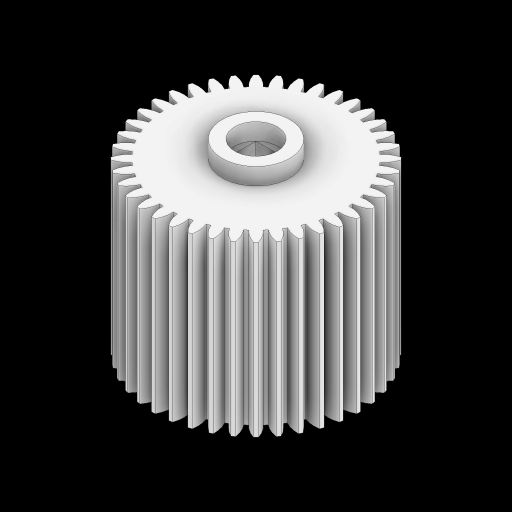
# Autodesk Inventor part: 피니언기어
Saved by Autodesk Inventor 2023 (Build 270158000, 158)
## iProperties
Created: 2024-07-04
Part Number: 피니언기어
Material: 일반
Document SubType Name: Modeling
Designer: OMS55
Density: 1 g/cm^3
Appearance: 기본값
Mass: 14.1026 g
Surface Area: 70.7702 cm^2
Volume: 14.1026 cm^3
Author: OMS55
Autodesk Inventor part; units mm, degrees
ref_plane "YZ Plane" through (0, 0, 0) normal (1, 0, 0) x (0, 1, 0)
ref_plane "XZ Plane" through (0, 0, 0) normal (0, 1, 0) x (-1, 0, 0)
ref_plane "XY Plane" through (0, 0, 0) normal (0, 0, 1) x (1, 0, 0)
sketch "스케치1" plane through (0, 0, 0) normal (0, 1, 0) x (-1, 0, 0)
  circle A0 centre (0, 0) radius 15.2
  arc A1 (12.978, 0.7559) -> (12.978, -0.7559) centre (0, 0) ccw
  line L0 (15.2, 0) -> (-15.2, 0) construction
  line L1 (15.1743, 0.8838) -> (-15.1743, -0.8838) construction
  line L2 (15.0972, 1.7646) -> (-15.0972, -1.7646) construction
  line L3 (14.9691, 2.6395) -> (-14.9691, -2.6395) construction
  line L4 (14.7903, 3.5054) -> (-14.7903, -3.5054) construction
  line L5 (14.5614, 4.3594) -> (-14.5614, -4.3594) construction
  line L6 (14.2833, 5.1987) -> (-14.2833, -5.1987) construction
  line L7 (13.9569, 6.0204) -> (-13.9569, -6.0204) construction
  line L8 (13.5832, 6.8217) -> (-13.5832, -6.8217) construction
  line L9 (13.1636, 7.6) -> (-13.1636, -7.6) construction
  line L10 (12.6994, 8.3525) -> (-12.6994, -8.3525) construction
  line L11 (12.1923, 9.0768) -> (-12.1923, -9.0768) construction
  line L12 (11.6439, 9.7704) -> (-11.6439, -9.7704) construction
  line L13 (11.0561, 10.4309) -> (-11.0561, -10.4309) construction
  line L14 (10.4309, 11.0561) -> (-10.4309, -11.0561) construction
  line L15 (9.7704, 11.6439) -> (-9.7704, -11.6439) construction
  line L16 (9.0768, 12.1923) -> (-9.0768, -12.1923) construction
  line L17 (8.3525, 12.6994) -> (-8.3525, -12.6994) construction
  line L18 (7.6, 13.1636) -> (-7.6, -13.1636) construction
  line L19 (6.8217, 13.5832) -> (-6.8217, -13.5832) construction
  line L20 (6.0204, 13.9569) -> (-6.0204, -13.9569) construction
  line L21 (5.1987, 14.2833) -> (-5.1987, -14.2833) construction
  line L22 (4.3594, 14.5614) -> (-4.3594, -14.5614) construction
  line L23 (3.5054, 14.7903) -> (-3.5054, -14.7903) construction
  line L24 (2.6395, 14.9691) -> (-2.6395, -14.9691) construction
  line L25 (1.7646, 15.0972) -> (-1.7646, -15.0972) construction
  line L26 (0.8838, 15.1743) -> (-0.8838, -15.1743) construction
  line L27 (0, 15.2) -> (0, -15.2) construction
  line L28 (-0.8838, 15.1743) -> (0.8838, -15.1743) construction
  line L29 (-1.7646, 15.0972) -> (1.7646, -15.0972) construction
  line L30 (-2.6395, 14.9691) -> (2.6395, -14.9691) construction
  line L31 (-3.5054, 14.7903) -> (3.5054, -14.7903) construction
  line L32 (-4.3594, 14.5614) -> (4.3594, -14.5614) construction
  line L33 (-5.1987, 14.2833) -> (5.1987, -14.2833) construction
  line L34 (-6.0204, 13.9569) -> (6.0204, -13.9569) construction
  line L35 (-6.8217, 13.5832) -> (6.8217, -13.5832) construction
  line L36 (-7.6, 13.1636) -> (7.6, -13.1636) construction
  line L37 (-8.3525, 12.6994) -> (8.3525, -12.6994) construction
  line L38 (-9.0768, 12.1923) -> (9.0768, -12.1923) construction
  line L39 (-9.7704, 11.6439) -> (9.7704, -11.6439) construction
  line L40 (-10.4309, 11.0561) -> (10.4309, -11.0561) construction
  line L41 (-11.0561, 10.4309) -> (11.0561, -10.4309) construction
  line L42 (-11.6439, 9.7704) -> (11.6439, -9.7704) construction
  line L43 (-12.1923, 9.0768) -> (12.1923, -9.0768) construction
  line L44 (-12.6994, 8.3525) -> (12.6994, -8.3525) construction
  line L45 (-13.1636, 7.6) -> (13.1636, -7.6) construction
  line L46 (-13.5832, 6.8217) -> (13.5832, -6.8217) construction
  line L47 (-13.9569, 6.0204) -> (13.9569, -6.0204) construction
  line L48 (-14.2833, 5.1987) -> (14.2833, -5.1987) construction
  line L49 (-14.5614, 4.3594) -> (14.5614, -4.3594) construction
  line L50 (-14.7903, 3.5054) -> (14.7903, -3.5054) construction
  line L51 (-14.9691, 2.6395) -> (14.9691, -2.6395) construction
  line L52 (-15.0972, 1.7646) -> (15.0972, -1.7646) construction
  line L53 (-15.1743, 0.8838) -> (15.1743, -0.8838) construction
  line L54 (-15.2, 0) -> (15.2, 0) construction
  line L55 (-15.1743, -0.8838) -> (15.1743, 0.8838) construction
  line L56 (-15.0972, -1.7646) -> (15.0972, 1.7646) construction
  line L57 (-14.9691, -2.6395) -> (14.9691, 2.6395) construction
  line L58 (-14.7903, -3.5054) -> (14.7903, 3.5054) construction
  line L59 (-14.5614, -4.3594) -> (14.5614, 4.3594) construction
  line L60 (-14.2833, -5.1987) -> (14.2833, 5.1987) construction
  line L61 (-13.9569, -6.0204) -> (13.9569, 6.0204) construction
  line L62 (-13.5832, -6.8217) -> (13.5832, 6.8217) construction
  line L63 (-13.1636, -7.6) -> (13.1636, 7.6) construction
  line L64 (-12.6994, -8.3525) -> (12.6994, 8.3525) construction
  line L65 (-12.1923, -9.0768) -> (12.1923, 9.0768) construction
  line L66 (-11.6439, -9.7704) -> (11.6439, 9.7704) construction
  line L67 (-11.0561, -10.4309) -> (11.0561, 10.4309) construction
  line L68 (-10.4309, -11.0561) -> (10.4309, 11.0561) construction
  line L69 (-9.7704, -11.6439) -> (9.7704, 11.6439) construction
  line L70 (-9.0768, -12.1923) -> (9.0768, 12.1923) construction
  line L71 (-8.3525, -12.6994) -> (8.3525, 12.6994) construction
  line L72 (-7.6, -13.1636) -> (7.6, 13.1636) construction
  line L73 (-6.8217, -13.5832) -> (6.8217, 13.5832) construction
  line L74 (-6.0204, -13.9569) -> (6.0204, 13.9569) construction
  line L75 (-5.1987, -14.2833) -> (5.1987, 14.2833) construction
  line L76 (-4.3594, -14.5614) -> (4.3594, 14.5614) construction
  line L77 (-3.5054, -14.7903) -> (3.5054, 14.7903) construction
  line L78 (-2.6395, -14.9691) -> (2.6395, 14.9691) construction
  line L79 (-1.7646, -15.0972) -> (1.7646, 15.0972) construction
  line L80 (-0.8838, -15.1743) -> (0.8838, 15.1743) construction
  line L81 (0, -15.2) -> (0, 15.2) construction
  line L82 (0.8838, -15.1743) -> (-0.8838, 15.1743) construction
  line L83 (1.7646, -15.0972) -> (-1.7646, 15.0972) construction
  line L84 (2.6395, -14.9691) -> (-2.6395, 14.9691) construction
  line L85 (3.5054, -14.7903) -> (-3.5054, 14.7903) construction
  line L86 (4.3594, -14.5614) -> (-4.3594, 14.5614) construction
  line L87 (5.1987, -14.2833) -> (-5.1987, 14.2833) construction
  line L88 (6.0204, -13.9569) -> (-6.0204, 13.9569) construction
  line L89 (6.8217, -13.5832) -> (-6.8217, 13.5832) construction
  line L90 (7.6, -13.1636) -> (-7.6, 13.1636) construction
  line L91 (8.3525, -12.6994) -> (-8.3525, 12.6994) construction
  line L92 (9.0768, -12.1923) -> (-9.0768, 12.1923) construction
  line L93 (9.7704, -11.6439) -> (-9.7704, 11.6439) construction
  line L94 (10.4309, -11.0561) -> (-10.4309, 11.0561) construction
  line L95 (11.0561, -10.4309) -> (-11.0561, 10.4309) construction
  line L96 (11.6439, -9.7704) -> (-11.6439, 9.7704) construction
  line L97 (12.1923, -9.0768) -> (-12.1923, 9.0768) construction
  line L98 (12.6994, -8.3525) -> (-12.6994, 8.3525) construction
  line L99 (13.1636, -7.6) -> (-13.1636, 7.6) construction
  line L100 (13.5832, -6.8217) -> (-13.5832, 6.8217) construction
  line L101 (13.9569, -6.0204) -> (-13.9569, 6.0204) construction
  line L102 (14.2833, -5.1987) -> (-14.2833, 5.1987) construction
  line L103 (14.5614, -4.3594) -> (-14.5614, 4.3594) construction
  line L104 (14.7903, -3.5054) -> (-14.7903, 3.5054) construction
  line L105 (14.9691, -2.6395) -> (-14.9691, 2.6395) construction
  line L106 (15.0972, -1.7646) -> (-15.0972, 1.7646) construction
  line L107 (15.1743, -0.8838) -> (-15.1743, 0.8838) construction
  arc A2 (15.1979, 0.25) -> (12.978, 0.7559) centre (13.2157, -3.3249) ccw
  arc A3 (12.978, -0.7559) -> (15.1979, -0.25) centre (13.2157, 3.3249) ccw
  dimension "d0" = 30.4
  dimension "d3" = 26
  dimension "d6" = 360
  dimension "d8" = 0.5
  dimension "d9" = 0.25
  constraints: 216 end point, 10 point on circle, 4 centre point, 3 point on line, 2 coincident, 2 tangent, 1 horizontal, 1 vertical alignment, 325 other
  measures "d0" diameter of A0
  measures "d3" diameter of A1
  measures "d8" distance of A3.end A2.start
  measures "d9" distance of A2.start L0.start
extrude "돌출1" add sketch "스케치1" along normal blind 25 contours A0 A3 A1 A2 picked at (-2.7443, 0.252)
pattern_circular "원형 패턴1" count 40 over 360 about axis through (0, 0, 0) along (0, 1, 0) of "돌출1"
sketch "스케치2" plane through (0, 25, 0) normal (0, 1, 0) x (1, 0, 0)
  circle A0 centre (0, 0) radius 3.15
  line L0 (-2.2274, 2.2274) -> (2.2274, 2.2274)
  line L1 (2.2274, 2.2274) -> (2.2274, -2.2274)
  line L2 (2.2274, -2.2274) -> (-2.2274, -2.2274)
  line L3 (-2.2274, -2.2274) -> (-2.2274, 2.2274)
  point P0 (-2.2274, 0)
  point P1 (0, 2.2274)
  dimension "d15" = 6.3
  dimension "d25" = 4.4548
  dimension "d26" = 4.4548
  constraints: 8 end point, 2 midpoint, 2 parallel, 1 centre point, 1 coincident, 1 horizontal, 1 horizontal alignment, 1 perpendicular, 1 vertical alignment
  measures "d15" diameter of A0
  measures "d25" distance of L0.start L0.end
  measures "d26" distance of L0.end L1.end
extrude "돌출2" cut sketch "스케치2" against normal blind 100 contours L1 L2 L3 L0
sketch "스케치3" plane through (0, 25, 0) normal (0, 1, 0) x (1, 0, 0)
  circle A0 centre (0, 0) radius 5
  circle A1 centre (0, 0) radius 3.15
  dimension "d18" = 10
  dimension "d19" = 6.3
  constraints: 2 centre point, 2 coincident
  measures "d18" diameter of A0
  measures "d19" diameter of A1
extrude "돌출3" add sketch "스케치3" along normal blind 2.5 and the other way blind 27.5
